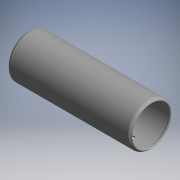
# Autodesk Inventor part: 04-2.2562C
Saved by Autodesk Inventor 2017.3 (Build 213256000, 256)
## iProperties
Part Number: 04-2.2562C
Material: Generic
Catalog Web Link: www.cadenas.de
Description: Tube-Original Line - Standard Air Cylinders
Vendor: BIMBA
Document SubType Name: Modeling
Designer: partserver
Manufacturer: BIMBA
Mass: 2.05875 g
Surface Area: 74.1623 cm^2
Volume: 2.05875 cm^3
Density: 1 g/cm^3
Appearance: PSOLRGB-180-180-180
Category: PARTsolutions
Company: BIMBA
Title: 04-2.2562C
Author: Cadenas PARTsolutions
Comments: Original Line - Standard Air Cylinders
PSOL_IDENT_0: {$CADENAS_DATA\23d-libs\bimba\bimba_brand\bimba_imperial\bimba_full_line\original_line_cylinders\sta
PSOL_IDENT_1: ndard_air_cylinders\tube.prj},199 {VTYP=3D},{NB=04-2.2562C},{LINA=04-2.2562C},{NN=Tube},{DATE=19.01.
PSOL_IDENT_2: 2022 10:19:38},{GEOMDATE=03.03.2020 12:52:40},{VERSION=},{LINEID=40},{WBVAR=MNT,ACTING,NR,L,FOURHOLE
PSOL_IDENT_3: S,SR,K},{WBNUMERIC=L,FOURHOLES}  {NB=04-2.2562C},{LINA=04-2.2562C},{KT=DUMMY},{PN=04-2.2562C},{BORE=
PSOL_IDENT_4: 0.75000000},{BOREPN=04},{MNT=},{MNTALG='' , 'Front Nose' , 'BF' , 'Front Block' , 'BFT' , 'Front Tru
PSOL_IDENT_5: nnion' , 'A' , 'Adjustable Stroke'},{ACTING=},{ACTINGALG= '' , 'Single Acting' , 'R' , 'Reverse/Doub
PSOL_IDENT_6: le Acting' },{NR=},{NRALG= '' , 'Without Non-rotating Rod' , 'NR' , 'With Non-rotating Rod' },{L=2.2
PSOL_IDENT_7: 560},{OD=0.8050},{ODN=0.8050},{ODP=0.8625},{ODB=0.8325},{ID=0.7615},{DV=0.00000000},{LV=0.00000000},
PSOL_IDENT_8: {LV1=0.00000000},{G=0.0300},{FOURHOLES=2},{AA=0.3750},{BB=0.0940},{SR=C},{SRALG= 'C' , 'Carbon Steel
PSOL_IDENT_9: Rod' , 'SR' , '303 Stainless Steel Rod' , '' , '303 Stainless Steel Rod'},{KALG= '', 'Standard' , '
PSOL_IDENT_10: K' , 'Ports Rotated 90deg' },{K=}
NB: 04-2.2562C
NN: Tube
NT: Original Line - Standard Air Cylinders
NBSYN: $PN.
LINA: 04-2.2562C
CATALOG: Bimba Products
BORE: 0
BOREPN: 04
MNT: Front Nose
MNTALG: '' , 'Front Nose' , 'BF' , 'Front Block' , 'BFT' , 'Front Trunnion' , 'A' , 'Adjustable Stroke'
ACTING: Single Acting
NR: Without Non-rotating Rod
L: 2.256
ODN: 0.805
ODP: 0.8625
ODB: 0.8325
ID: 0.7615
DV: 0
LV: 0
LV1: 0
G: 0.03
FOURHOLES: 2
AA: 0.375
BB: 0.094
SR: Carbon Steel Rod
K: Standard
SUPPLIER: BIMBA
ARTICLENO: 04-2.2562C
BOMINFO: 04-2.2562C
CREATOR: CADENAS GmbH
Autodesk Inventor part; units mm, degrees
ref_plane "YZ Plane" through (0, 0, 0) normal (1, 0, 0) x (0, 1, 0)
ref_plane "XZ Plane" through (0, 0, 0) normal (0, 1, 0) x (-1, 0, 0)
ref_plane "XY Plane" through (0, 0, 0) normal (0, 0, 1) x (1, 0, 0)
sketch "Sketch_1" plane through (0, 0, 0) normal (0, 0, 1) x (1, 0, 0)
  line L0 (57.3024, 0) -> (0, 0)
  arc A0 (-0.6395, 9.3472) -> (-0.6395, 9.1676) centre (-0.5497, 9.2574) ccw
  line L1 (-0.6395, 9.1676) -> (-0.381, 8.9091)
  line L2 (-0.381, 8.9091) -> (0, 8.9091)
  line L3 (0, 8.9091) -> (0.762, 9.671)
  line L4 (0.762, 9.671) -> (56.5404, 9.671)
  line L5 (56.5404, 9.671) -> (57.3024, 8.9091)
  line L6 (57.3024, 8.9091) -> (57.6834, 8.9091)
  line L7 (57.6834, 8.9091) -> (57.9419, 9.1676)
  arc A1 (57.9419, 9.1676) -> (57.9419, 9.3472) centre (57.8521, 9.2574) ccw
  line L8 (57.9419, 9.3472) -> (57.2888, 10.0003)
  arc A2 (57.2888, 10.0003) -> (56.7499, 10.2235) centre (56.75, 9.4615) ccw
  line L9 (56.7499, 10.2235) -> (0.5524, 10.2235)
  arc A3 (0.5524, 10.2235) -> (0.0136, 10.0003) centre (0.5524, 9.4615) ccw
  line L10 (0.0136, 10.0003) -> (-0.6395, 9.3472)
  constraints: 22 end point, 8 point on circle, 4 centre point
revolve "Revolution1" add sketch "Sketch_1" angle 360 about axis through (57.3024, 0, 0) along (1, 0, 0)
sketch "Sketch_4" plane through (0, 0, 0) normal (0, 0, 1) x (1, 0, 0)
  circle A0 centre (8.763, 0) radius 1.1938
  constraints: 1 centre point
extrude "Extrusion1" cut sketch "Sketch_4" along normal blind 10.2235
ref_plane "cp1_XY" through (28.6512, 0, 10.2235) normal (1, 0, 0) x (0, 0, -1)
ref_plane "cp1_YZ" through (28.6512, 0, 10.2235) normal (0, 0, -1) x (0, 1, 0)
ref_plane "cp1_ZX" through (28.6512, 0, 10.2235) normal (0, 1, 0) x (1, 0, 0)
ref_plane "cp2_XY" through (28.6512, 10.2235, 0) normal (1, 0, 0) x (0, 0, -1)
ref_plane "cp2_YZ" through (28.6512, 10.2235, 0) normal (0, 0, -1) x (0, 1, 0)
ref_plane "cp2_ZX" through (28.6512, 10.2235, 0) normal (0, 1, 0) x (1, 0, 0)
ref_plane "cp3_XY" through (28.6512, 0, -10.2235) normal (1, 0, 0) x (0, 0, -1)
ref_plane "cp3_YZ" through (28.6512, 0, -10.2235) normal (0, 0, -1) x (0, 1, 0)
ref_plane "cp3_ZX" through (28.6512, 0, -10.2235) normal (0, 1, 0) x (1, 0, 0)
ref_plane "cp4_XY" through (28.6512, -10.2235, 0) normal (1, 0, 0) x (0, 0, -1)
ref_plane "cp4_YZ" through (28.6512, -10.2235, 0) normal (0, 0, -1) x (0, 1, 0)
ref_plane "cp4_ZX" through (28.6512, -10.2235, 0) normal (0, 1, 0) x (1, 0, 0)
ref_plane "tube_front_XY" through (0, 0, 0) normal (1, 0, 0) x (0, 0, -1)
ref_plane "tube_front_YZ" through (0, 0, 0) normal (0, 0, -1) x (0, 1, 0)
ref_plane "tube_front_ZX" through (0, 0, 0) normal (0, 1, 0) x (1, 0, 0)
ref_plane "tube_rear_XY" through (57.3024, 0, 0) normal (1, 0, 0) x (0, 0, -1)
ref_plane "tube_rear_YZ" through (57.3024, 0, 0) normal (0, 0, -1) x (0, 1, 0)
ref_plane "tube_rear_ZX" through (57.3024, 0, 0) normal (0, 1, 0) x (1, 0, 0)
body "Solid1"
